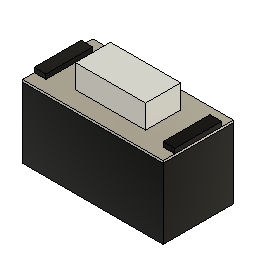
ver4-0420 (Autodesk Fusion 360 archive; units mm, degrees)
design "SW_タクト"
Autodesk Fusion 360 part; units mm, degrees
sketch "スケッチ1" plane through (0, 0, 0) normal (0, 0, 1) x (1, 0, 0)
  line L0 (3, 1.5) -> (-3, 1.5)
  line L1 (-3, 1.5) -> (-3, -1.5)
  line L2 (-3, -1.5) -> (3, -1.5)
  line L3 (3, -1.5) -> (3, 1.5)
  line L4 (3, 1.5) -> (-3, -1.5) construction
  line L5 (-3, 1.5) -> (3, -1.5) construction
  dimension "d1" = 6
  dimension "d2" = 3
  constraint horizontal L0
  constraint perpendicular L0 L1
  constraint parallel L0 L2
  constraint parallel L1 L3
  constraint coincident L4 origin
  constraint coincident L5 origin
  measures "d1" distance of L1.end L2.end
  measures "d2" distance of L0.end L1.end
extrude "押し出し1" add sketch "スケッチ1" along normal blind 3 makes body 1
sketch "スケッチ2" plane through (0, 0, 3) normal (0, 0, 1) x (-1, 0, 0)
  line L0 (-3, 1.5) -> (-3, -1.5)
  line L1 (-3, -1.5) -> (3, -1.5)
  line L2 (3, -1.5) -> (3, 1.5)
  line L3 (3, 1.5) -> (-3, 1.5)
extrude "押し出し2" add sketch "スケッチ2" along normal blind 0.1 separate body makes body 2
sketch "スケッチ3" plane through (0, 0, 3.1) normal (0, 0, 1) x (-1, 0, 0)
  line L0 (3, 1.5) -> (-3, 1.5)
  line L1 (-3, 1.5) -> (-3, -1.5)
  line L2 (-3, -1.5) -> (3, -1.5)
  line L3 (3, -1.5) -> (3, 1.5)
  line L4 (-1.5, 0.75) -> (1.5, 0.75)
  line L5 (1.5, 0.75) -> (1.5, -0.75)
  line L6 (1.5, -0.75) -> (-1.5, -0.75)
  line L7 (-1.5, -0.75) -> (-1.5, 0.75)
  line L8 (-1.5, 0.75) -> (1.5, -0.75) construction
  line L9 (1.5, 0.75) -> (-1.5, -0.75) construction
  line L10 (3, 0) -> (3, -1)
  line L11 (3, -1) -> (2.5, -1)
  line L12 (2.5, -1) -> (2.5, 1)
  line L13 (2.5, 1) -> (3, 1)
  line L14 (3, 0) -> (3, 1)
  line L15 (-3, 0) -> (-3, 1)
  line L16 (-3, 0) -> (-3, -1)
  line L17 (-3, -1) -> (-2.5, -1)
  line L18 (-2.5, 1) -> (-3, 1)
  line L19 (-2.5, -1) -> (-2.5, 1)
  dimension "d7" = 3
  dimension "d8" = 1.5
  dimension "d11" = 1
  dimension "d12" = 0.5
  dimension "d13" = 2
  constraint horizontal L4
  constraint perpendicular L4 L5
  constraint parallel L4 L6
  constraint parallel L5 L7
  constraint coincident L8 origin
  constraint coincident L9 origin
  constraint midpoint L3 L10.start
  constraint parallel L3 L10
  constraint perpendicular L10 L11
  constraint perpendicular L11 L12
  constraint perpendicular L12 L13
  constraint perpendicular L13 L14
  measures "d7" distance of L5.end L6.end
  measures "d8" distance of L4.end L5.end
  measures "d11" distance of L10.start L10.end
  measures "d12" distance of L10.end L11.end
  measures "d13" distance of L11.end L12.end
extrude "押し出し3" add sketch "スケッチ3" along normal blind 1 separate body contours L4 L5 L6 L7 makes body 3
extrude "押し出し4" add sketch "スケッチ3" along normal blind 0.2 separate body contours L3 L10 L11 L12 L13 L14 | L1 L15 L16 L17 L18 L19 makes body 4 at (-2.6667, -0.3333, 3.1) makes body 5 at (2.8333, -0.3333, 3.1)

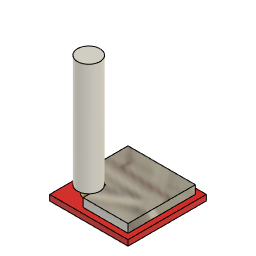
design "TWE-Lite-RED"
Autodesk Fusion 360 part; units mm, degrees
sketch "スケッチ1" plane through (0, 0, 0) normal (0, 0, 1) x (1, 0, 0)
  line L0 (6.985, -6.985) -> (-6.985, -6.985)
  line L1 (-6.985, -6.985) -> (-6.985, 6.985)
  line L2 (-6.985, 6.985) -> (6.985, 6.985)
  line L3 (6.985, 6.985) -> (6.985, -6.985)
  line L4 (6.985, -6.985) -> (-6.985, 6.985) construction
  line L5 (-6.985, -6.985) -> (6.985, 6.985) construction
  dimension "d1" = 13.97
  dimension "d2" = 13.97
  constraint horizontal L0
  constraint perpendicular L0 L1
  constraint parallel L0 L2
  constraint parallel L1 L3
  constraint coincident L4 origin
  constraint coincident L5 origin
  measures "d1" distance of L1.end L2.end
  measures "d2" distance of L0.end L1.end
extrude "押し出し1" add sketch "スケッチ1" along normal blind 1 makes body 1
sketch "スケッチ2" plane through (0, 0, 1) normal (0, 0, 1) x (-1, 0, 0)
  line L0 (-6.985, -6.985) -> (6.985, -6.985)
  line L1 (6.985, -6.985) -> (6.985, 6.985)
  line L2 (6.985, 6.985) -> (-6.985, 6.985)
  line L3 (-6.985, 6.985) -> (-6.985, -6.985)
  line L4 (6, 6) -> (-6, 6)
  line L5 (-6, 6) -> (-6, -6)
  line L6 (-6, -6) -> (6, -6)
  line L7 (6, -6) -> (6, 6)
  line L8 (6, 6) -> (2, 6)
  line L9 (2, 6) -> (2, 2)
  line L10 (2, 2) -> (6, 2)
  line L11 (6, 2) -> (6, 6)
  circle A0 centre (3.5, 3.5) radius 1
  circle A1 centre (3.5, 3.5) radius 0.9
  dimension "d5" = 12
  dimension "d6" = 12
  dimension "d7" = 4
  dimension "d8" = 4
  dimension "d13" = 2
  dimension "d14" = -0.1
  constraint horizontal L4
  constraint perpendicular L4 L5
  constraint parallel L4 L6
  constraint parallel L5 L7
  constraint horizontal L8
  constraint vertical L9
  constraint horizontal L10
  constraint vertical L11
  measures "d5" distance of L5.end L6.end
  measures "d6" distance of L4.end L5.end
  measures "d7" distance of L4.start L8.end
  measures "d8" distance of L4.start L10.end
  measures "d13" diameter of A0
extrude "押し出し2" add sketch "スケッチ2" along normal blind 1.5 separate body contours L4 L5 L6 L7 L9 L10 makes body 2
extrude "押し出し3" add sketch "スケッチ2" along normal blind 1.5 separate body contours A0 makes body 3
sketch "スケッチ3" plane through (0, 0, 2.5) normal (0, 0, 1) x (-1, 0, 0)
  circle A0 centre (3.5, 3.5) radius 0.9
  circle A1 centre (3.5, 3.5) radius 1
  circle A2 centre (3.5, 3.5) radius 2
  dimension "d17" = 4
  constraint concentric A0 A2
  measures "d17" diameter of A2
extrude "押し出し4" add sketch "スケッチ3" along normal blind 20 separate body contours A0 | A1 | A2 makes body 4

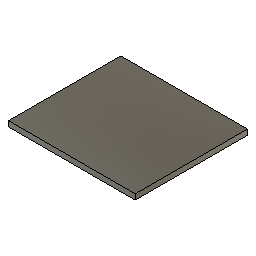
design "GPS仮"
Autodesk Fusion 360 part; units mm, degrees
sketch "スケッチ1" plane through (0, 0, 0) normal (0, 0, 1) x (1, 0, 0)
  line L0 (-17.5, -15.5) -> (17.5, -15.5)
  line L1 (17.5, -15.5) -> (17.5, 15.5)
  line L2 (17.5, 15.5) -> (-17.5, 15.5)
  line L3 (-17.5, 15.5) -> (-17.5, -15.5)
  line L4 (-17.5, -15.5) -> (17.5, 15.5) construction
  line L5 (17.5, -15.5) -> (-17.5, 15.5) construction
  dimension "d1" = 35
  dimension "d2" = 31
  constraint horizontal L0
  constraint perpendicular L0 L1
  constraint parallel L0 L2
  constraint parallel L1 L3
  constraint coincident L4 origin
  constraint coincident L5 origin
  measures "d1" distance of L1.end L2.end
  measures "d2" distance of L0.end L1.end
extrude "押し出し1" add sketch "スケッチ1" along normal blind 1.5

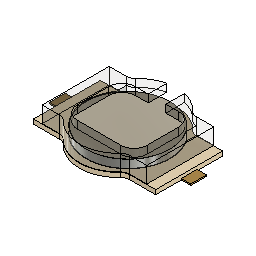
design "C2032 & its-cover"
Autodesk Fusion 360 part; units mm, degrees
sketch "スケッチ1" plane through (0, 0, 0) normal (0, 0, 1) x (1, 0, 0)
  line L0 (-13.845, -7.58) -> (-13.845, 7.58)
  line L1 (13.845, 7.58) -> (13.845, -7.58)
  line L2 (-16, 1.78) -> (-16, -1.78)
  line L3 (16, -1.78) -> (16, 1.78)
  line L4 (-13.845, -1.78) -> (-16, -1.78)
  line L5 (-13.845, 1.78) -> (-16, 1.78)
  line L6 (13.845, 1.78) -> (16, 1.78)
  line L7 (13.845, -1.78) -> (16, -1.78)
  arc A0 (-6.4609, -8.209) -> (0, -11) centre (0, -2.1263) ccw
  arc A1 (0, -11) -> (6.4609, -8.209) centre (0, -2.1263) ccw
  arc A2 (6.4609, 8.209) -> (0, 11) centre (0, 2.1263) ccw
  arc A3 (0, 11) -> (-6.4609, 8.209) centre (0, 2.1263) ccw
  line L8 (-13.845, 7.58) -> (-7.9171, 7.58)
  line L9 (7.9171, 7.58) -> (13.845, 7.58)
  line L10 (13.845, -7.58) -> (7.9171, -7.58)
  line L11 (-7.9171, -7.58) -> (-13.845, -7.58)
  arc A4 (-7.9171, 7.58) -> (-6.4609, 8.209) centre (-7.9171, 9.58) ccw
  arc A5 (6.4609, 8.209) -> (7.9171, 7.58) centre (7.9171, 9.58) ccw
  arc A6 (7.9171, -7.58) -> (6.4609, -8.209) centre (7.9171, -9.58) ccw
  arc A7 (-6.4609, -8.209) -> (-7.9171, -7.58) centre (-7.9171, -9.58) ccw
  dimension "d6" = 27.69
  dimension "d7" = 15.16
  dimension "d15" = 2
  constraint horizontal L10
  constraint perpendicular L0 L10
  constraint parallel L8 L10
  constraint parallel L0 L1
  constraint parallel L2 L3
  constraint collinear L8 L9
  constraint collinear L10 L11
  constraint tangent A3 A4
  constraint tangent L8 A4
  constraint tangent A2 A5
  constraint tangent L9 A5
  constraint equal A4 A5
  constraint tangent A1 A6
  constraint tangent L10 A6
  constraint equal A4 A6
  constraint tangent A0 A7
  constraint tangent L11 A7
  constraint equal A4 A7
  measures "d6" distance of L0.end L1.start
  measures "d7" distance of L0.start L0.end
  measures "d15" radius of A4
extrude "押し出し1" add sketch "スケッチ1" along normal blind 1 contours L0 L1 A0 A1 A2 A3 L8 L9 L10 L11 A4 A5 A6 A7 makes body 1
extrude "押し出し2" add sketch "スケッチ1" along normal blind 0.3 contours L0 L2 L4 L5 | L1 L3 L6 L7 bodies 1
sketch "スケッチ2" plane through (0, 0, 1) normal (0, 0, 1) x (-1, 0, 0)
  arc A0 (6.4609, 8.209) -> (-6.4609, 8.209) centre (0, 2.1263) ccw
  arc A1 (-7.9171, 7.58) -> (-6.4609, 8.209) centre (-7.9171, 9.58) ccw
  line L0 (-7.9171, 7.58) -> (-13.845, 7.58)
  line L1 (-13.845, 7.58) -> (-13.845, -7.58)
  line L2 (-13.845, -7.58) -> (-7.9171, -7.58)
  arc A2 (-6.4609, -8.209) -> (-7.9171, -7.58) centre (-7.9171, -9.58) ccw
  arc A3 (-6.4609, -8.209) -> (6.4609, -8.209) centre (0, -2.1263) ccw
  arc A4 (7.9171, -7.58) -> (6.4609, -8.209) centre (7.9171, -9.58) ccw
  line L3 (7.9171, -7.58) -> (13.845, -7.58)
  line L4 (13.845, -7.58) -> (13.845, 7.58)
  line L5 (13.845, 7.58) -> (7.9171, 7.58)
  arc A5 (6.4609, 8.209) -> (7.9171, 7.58) centre (7.9171, 9.58) ccw
  line L6 (4.9171, 6.58) -> (-4.9171, 6.58)
  line L7 (-7.9171, 3.58) -> (-7.9171, -3.58)
  line L8 (-4.9171, -6.58) -> (4.9171, -6.58)
  line L9 (7.9171, -3.58) -> (7.9171, 3.58)
  arc A6 (4.9171, -6.58) -> (7.9171, -3.58) centre (4.9171, -3.58) ccw
  arc A7 (-7.9171, -3.58) -> (-4.9171, -6.58) centre (-4.9171, -3.58) ccw
  arc A8 (-4.9171, 6.58) -> (-7.9171, 3.58) centre (-4.9171, 3.58) ccw
  arc A9 (7.9171, 3.58) -> (4.9171, 6.58) centre (4.9171, 3.58) ccw
  line L10 (11.845, -7.58) -> (11.845, 7.58)
  line L11 (-11.845, 7.58) -> (-11.845, -7.58)
  line L12 (7.9171, -7.58) -> (7.9171, -3.58)
  line L13 (-7.9171, -7.58) -> (-7.9171, -3.58)
  line L14 (2, -10.7717) -> (2, -6.58)
  line L15 (-2, -10.7717) -> (-2, -6.58)
  circle A10 centre (0, 0) radius 9.5
  dimension "d21" = 3
  dimension "d22" = -2
  dimension "d23" = -2
  dimension "d28" = 19
  constraint horizontal L6
  constraint perpendicular L6 L7
  constraint parallel L6 L8
  constraint parallel L7 L9
  constraint tangent L8 A6
  constraint tangent L9 A6
  constraint tangent L7 A7
  constraint tangent L8 A7
  constraint equal A6 A7
  constraint tangent L6 A8
  constraint tangent L7 A8
  constraint equal A6 A8
  constraint tangent L6 A9
  constraint tangent L9 A9
  constraint equal A6 A9
  constraint tangent A6 L12
  constraint tangent A7 L13
  constraint coincident A3 L14.start
  constraint coincident A3 L15.start
  constraint coincident A10.centre origin
  measures "d21" radius of A6
  measures "d28" diameter of A10
extrude "押し出し3" add sketch "スケッチ2" along normal blind 3.75 and the other way blind -0.1 separate body contours A0 A1 L0 L2 L3 L5 A5 L10 L11 L12 L13 A10 | A3 A4 L12 L14 A10 | A2 A3 L13 L15 A10 | L8 A6 L12 L14 A10 | L6 L7 L9 A8 A9 L12 L13 A10 | L8 A7 L13 L15 A10 makes body 2
extrude "押し出し4" cut sketch "スケッチ2" along normal blind 2 contours A3 A4 L12 L14 A10 | A2 A3 L13 L15 A10 | L8 A6 L12 L14 A10 | L6 L7 L9 A8 A9 L12 L13 A10 | L8 A7 L13 L15 A10 | L8 L14 L15 A10 bodies 2
sketch "スケッチ3" plane through (0, 0, 1) normal (0, 0, 1) x (-1, 0, 0)
  arc A0 (6.4609, 8.209) -> (-6.4609, 8.209) centre (0, 2.1263) ccw
  arc A1 (-7.9171, 7.58) -> (-6.4609, 8.209) centre (-7.9171, 9.58) ccw
  line L0 (-7.9171, 7.58) -> (-13.845, 7.58)
  line L1 (-13.845, 7.58) -> (-13.845, -7.58)
  line L2 (-13.845, -7.58) -> (-7.9171, -7.58)
  arc A2 (-6.4609, -8.209) -> (-7.9171, -7.58) centre (-7.9171, -9.58) ccw
  arc A3 (-6.4609, -8.209) -> (6.4609, -8.209) centre (0, -2.1263) ccw
  arc A4 (7.9171, -7.58) -> (6.4609, -8.209) centre (7.9171, -9.58) ccw
  line L3 (7.9171, -7.58) -> (13.845, -7.58)
  line L4 (13.845, -7.58) -> (13.845, 7.58)
  line L5 (13.845, 7.58) -> (7.9171, 7.58)
  arc A5 (6.4609, 8.209) -> (7.9171, 7.58) centre (7.9171, 9.58) ccw
  circle A6 centre (0, 0) radius 9.5
  circle A7 centre (0, 0) radius 9.4
  dimension "d39" = 18.8
  constraint coincident A6.centre A7.centre
  measures "d39" diameter of A7
extrude "押し出し7" add sketch "スケッチ3" along normal blind 1.9 and the other way blind -0.1 separate body contours A7 makes body 3
equation "d26 = 4.75 mm - 1 mm"
equation "d28 = 22.000 mm - 3 mm"
equation "d39 = 19 mm - 0.1 mm - 0.1 mm"
equation "d44 = 2 mm - 0.1 mm"
named bodies: "mount", "cover", "C2032"
